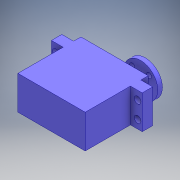
# Autodesk Inventor part: MG996 伺服馬達
Saved by Autodesk Inventor 2017 (Build 210142000, 142)
## iProperties
Part Number: MG996 伺服馬達
Material: 一般
Document SubType Name: Modeling
Designer: Brian
Density: 2.02898 g/cm^3
Appearance: 預設(2)
Mass: 65 g
Surface Area: 78.7048 cm^2
Volume: 32.0359 cm^3
Author: Brian
Autodesk Inventor part; units mm, degrees
ref_plane "YZ Plane" through (0, 0, 0) normal (1, 0, 0) x (0, 1, 0)
ref_plane "XZ Plane" through (0, 0, 0) normal (0, 1, 0) x (-1, 0, 0)
ref_plane "XY Plane" through (0, 0, 0) normal (0, 0, 1) x (1, 0, 0)
sketch "草圖1" plane through (0, 0, 0) normal (0, 0, 1) x (1, 0, 0)
  line L0 (0, 0) -> (40, 0)
  line L1 (40, 0) -> (40, 37.5)
  line L2 (40, 37.5) -> (0, 37.5)
  line L3 (0, 37.5) -> (0, 0)
  dimension "d0" = 37.5
  dimension "d1" = 40
  constraints: 8 end point, 2 parallel, 1 horizontal, 1 perpendicular
  measures "d0" distance of L2.end L0.start
  measures "d1" distance of L0.start L0.end
extrude "擠出1" add sketch "草圖1" along normal mid plane 20
sketch "草圖2" plane through (0, 0, 10) normal (0, 0, 1) x (1, 0, 0)
  line L0 (-7, 31.9) -> (47, 31.9)
  line L1 (47, 31.9) -> (47, 26.9)
  line L2 (47, 26.9) -> (-7, 26.9)
  line L3 (-7, 26.9) -> (-7, 31.9)
  line L4 (0, 37.5) -> (0, 0) projected
  line L5 (0, 0) -> (40, 0) projected
  dimension "d4" = 54
  dimension "d5" = 7
  dimension "d6" = 26.9
  dimension "d7" = 5
  constraints: 8 end point, 2 parallel, 1 horizontal, 1 perpendicular
  measures "d4" distance between parallel lines of L1 L3
  measures "d5" distance between parallel lines of L4 L3
  measures "d6" distance between parallel lines of L5 L2
  measures "d7" distance of L0.end L1.end
extrude "擠出2" add sketch "草圖2" against normal blind 20
sketch "草圖3" plane through (-7, 31.9, 10) normal (0, 1, 0) x (1, 0, 0)
  line L0 (2.7, 15) -> (51.3, 15)
  line L1 (51.3, 15) -> (51.3, 5)
  line L2 (51.3, 5) -> (2.7, 5)
  line L3 (2.7, 5) -> (2.7, 15)
  line L4 (47, 20) -> (54, 20) projected
  line L5 (54, 0) -> (54, 20) projected
  circle A0 centre (2.7, 15) radius 2
  circle A1 centre (2.7, 5) radius 2
  circle A2 centre (51.3, 5) radius 2
  circle A3 centre (51.3, 15) radius 2
  point P0 (7, 10)
  dimension "d10" = 10
  dimension "d11" = 5
  dimension "d12" = 2.7
  dimension "d13" = 48.6
  dimension "d14" = 4
  constraints: 8 end point, 4 centre point, 4 coincident, 3 equal radius, 2 parallel, 1 horizontal, 1 perpendicular
  measures "d10" distance of L0.end L1.end
  measures "d11" distance between parallel lines of L4 L0
  measures "d12" distance between parallel lines of L5 L1
  measures "d13" distance of L1.end L2.end
  measures "d14" diameter of A3
extrude "擠出3" cut sketch "草圖3" against normal blind 20 contours L3 A0 L0 | L0 A0 L3 | A3 L1 L0 | L0 L1 A3 | A1 L2 L3 | L3 L2 A1 | A2 L2 L1 | L1 L2 A2
sketch "草圖4" plane through (0, 0, 0) normal (0, 0, 1) x (1, 0, 0)
  line L0 (0, 37.5) -> (40, 37.5) projected
  line L1 (32, 37.5) -> (30, 37.5)
  line L2 (30, 37.5) -> (30, 45.7)
  line L3 (30, 45.7) -> (32, 45.7)
  line L4 (32, 45.7) -> (32, 37.5)
  line L5 (-2.3, 26.9) -> (-6.3, 26.9) projected
  line L6 (-6.3, 31.9) -> (-2.3, 31.9) projected
  line L7 (-4.3, 26.9) -> (-4.3, 31.9)
  line L8 (40, 0) -> (0, 0) projected
  line L9 (30, 45.7) -> (40.2, 45.7)
  line L10 (40.2, 45.7) -> (40.2, 42.9583)
  line L11 (40.2, 42.9583) -> (30, 42.9583)
  line L12 (30, 42.9583) -> (30, 45.7)
  dimension "d17" = 34.3
  dimension "d18" = 45.7
  dimension "d19" = 2
  dimension "d20" = 10.2
  constraints: 18 end point, 4 parallel, 2 horizontal, 2 midpoint, 2 perpendicular, 1 point on line
  measures "d17" distance between parallel lines of L2 L7
  measures "d18" distance between parallel lines of L8 L3
  measures "d19" distance of L2.end L3.end
  measures "d20" distance of L2.end L9.end
revolve "迴轉1" add sketch "草圖4" angle 360 about axis through (30, 37.5, 0) along (0, 1, 0)
sketch "草圖5" plane through (30, 45.7, 0) normal (0, 1, 0) x (1, 0, 0)
  line L0 (-4.9497, -4.9497) -> (4.9497, -4.9497)
  line L1 (4.9497, -4.9497) -> (4.9497, 4.9497)
  line L2 (4.9497, 4.9497) -> (-4.9497, 4.9497)
  line L3 (-4.9497, 4.9497) -> (-4.9497, -4.9497)
  line L4 (-4.9497, -4.9497) -> (4.9497, 4.9497) construction
  line L5 (4.9497, -4.9497) -> (-4.9497, 4.9497) construction
  circle A0 centre (0, 0) radius 10.2 projected
  point P0 (-30, 0)
  point P1 (0, 0)
  dimension "d22" = 14
  constraints: 12 end point, 3 midpoint, 2 parallel, 2 perpendicular, 1 coincident, 1 horizontal
  measures "d22" distance of L0.start L1.end
hole "孔1" at (34.9497, 45.7, -4.9497) at (34.9497, 45.7, 4.9497) at (25.0503, 45.7, 4.9497) at (25.0503, 45.7, -4.9497) direction (0, -1, 0) diameter 3 depth 4 tip angle 118
move faces "移動1" translate (0, 1.2, 0) faces at (-0.786, 31.9, -1.5071)
move faces "移動2" translate (0, 1.2, 0) faces at (40.786, 31.9, 1.5071)
